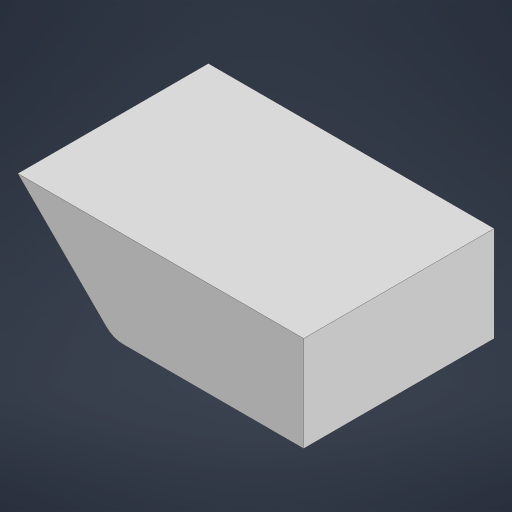
# Autodesk Inventor part: Hard_Stop
Saved by Autodesk Inventor 2023 (Build 270158000, 158)
## iProperties
Created: 2024-02-23
Part Number: Hard_Stop
Material: Generic
Document SubType Name: Modeling
Designer: kelle
Density: 1 g/cm^3
Appearance: Default
Author: kelle
Autodesk Inventor part; units mm, degrees
ref_plane "YZ Plane" through (0, 0, 0) normal (1, 0, 0) x (0, 1, 0)
ref_plane "XZ Plane" through (0, 0, 0) normal (0, 1, 0) x (-1, 0, 0)
ref_plane "XY Plane" through (0, 0, 0) normal (0, 0, 1) x (1, 0, 0)
sketch "Sketch1" plane through (0, 0, 0) normal (0, 0, 1) x (1, 0, 0)
  line L0 (19.05, -6.35) -> (-19.05, -6.35)
  line L1 (-19.05, -6.35) -> (-19.05, 6.35)
  line L2 (-19.05, 6.35) -> (19.05, 6.35)
  line L3 (19.05, 6.35) -> (19.05, -6.35)
  line L4 (19.05, -6.35) -> (-19.05, 6.35) construction
  line L5 (-19.05, -6.35) -> (19.05, 6.35) construction
  line L6 (-19.05, 6.35) -> (-6.35, -6.35)
  line L7 (-19.05, 6.35) -> (1.6336, 6.35) construction
  point P0 (0, 0)
  dimension "d0" = 38.1
  dimension "d1" = 12.7
  dimension "d2" = 45
  constraints: 16 end point, 2 horizontal, 2 midpoint, 2 parallel, 1 perpendicular, 1 point on line
  measures "d0" distance of L1.end L2.end
  measures "d1" distance of L0.end L1.end
  measures "d2" angle of L6 L7
extrude "Extrusion1" add sketch "Sketch1" along normal blind 25.4 contours L0 L6 L2 L3
fillet "Fillet1" radius 3.175 1 edges at (-6.35, -6.35, 12.7)
body "Solid1"
